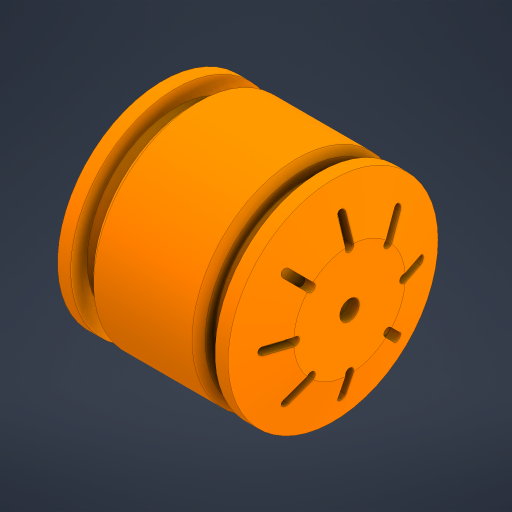
# Autodesk Inventor part: wheel
Saved by Autodesk Inventor 2024 (Build 280153000, 153)
## iProperties
Created: 2023-09-26
Part Number: wheel
Material: Типовые
Document SubType Name: Modeling
Designer: user
Density: 1 g/cm^3
Appearance: По умолчанию
Mass: 47.7551 g
Surface Area: 315.947 cm^2
Volume: 47.7551 cm^3
Author: user
Autodesk Inventor part; units mm, degrees
ref_plane "YZ Plane" through (0, 0, 0) normal (1, 0, 0) x (0, 1, 0)
ref_plane "XZ Plane" through (0, 0, 0) normal (0, 1, 0) x (-1, 0, 0)
sketch "Эскиз1" plane through (0, 0, 0) normal (0, 0, 1) x (1, 0, 0)
  line L0 (0, 0) -> (0, 32)
  line L1 (0, 32) -> (4, 32)
  line L2 (4, 32) -> (4, 27)
  line L3 (4, 27) -> (9, 27)
  line L4 (9, 27) -> (9, 32)
  line L5 (9, 32) -> (43, 32)
  line L6 (43, 32) -> (43, 27)
  line L7 (43, 27) -> (48, 27)
  line L8 (48, 27) -> (48, 32)
  line L9 (48, 32) -> (52, 32)
  line L10 (52, 32) -> (52, 0)
  line L11 (52, 0) -> (0, 0)
  dimension "d0" = 32
  dimension "d1" = 27
  dimension "d2" = 5
  dimension "d3" = 34
  dimension "d4" = 4
  constraints: 24 end point, 8 perpendicular, 6 point on line, 2 collinear, 1 vertical
  measures "d0" distance of L0.start L0.end
  measures "d1" vertical distance of L0.start L2.end
  measures "d2" distance of L2.end L3.end
  measures "d3" distance of L4.end L5.end
  measures "d4" distance of L0.end L1.end
revolve "Вращение1" add sketch "Эскиз1" angle 360 about axis through (52, 0, 0) along (-1, 0, 0)
sketch "Эскиз2" plane through (0, 0, 0) normal (0, 0, 1) x (1, 0, 0)
  line L0 (52, 32) -> (52, -32) projected
  line L1 (52, 32) -> (57, 17)
  line L2 (52, 0) -> (57, 0)
  line L3 (57, 0) -> (57, 17)
  point P0 (0, 0)
  dimension "d6" = 17
  dimension "d7" = 5
  constraints: 6 end point, 1 horizontal, 1 midpoint, 1 perpendicular
  measures "d6" distance of L2.end L1.end
  measures "d7" distance of L2.start L2.end
revolve "Вращение2" add sketch "Эскиз2" angle 360 about axis through (52, 0, 0) along (1, 0, 0)
shell "Оболочка1" thickness 3 removed faces 1 at (0, 9.4449, -4.957)
ref_plane "РабПлоскость1" through (26, 0, -32) normal (0, 0, 1) x (1, 0, 0)
chamfer "Фаска1" distance 2 angle 45 2 edges at (9, -32, 0) (43, -32, 0)
sketch "Эскиз9" plane through (57, 0, 0) normal (1, 0, 0) x (0, 0, -1)
  circle A0 centre (0, 0) radius 3
  dimension "d68" = 6
  constraints: 1 centre point, 1 coincident
  measures "d68" diameter of A0
extrude "Выдавливание6" cut sketch "Эскиз9" against normal through all
sketch "Эскиз21" plane through (54, 0, 0) normal (-1, 0, 0) x (0, 0, 1)
  circle A0 centre (0, 0) radius 3 projected
  circle A1 centre (0, 0) radius 16.5132 projected
extrude "Выдавливание17" add sketch "Эскиз21" along normal blind 0.1
sketch "Эскиз22" plane through (53.9, 0, 0) normal (-1, 0, 0) x (0, 0, 1)
  line L0 (-3.4641, -6) -> (3.4641, -6) projected
  line L1 (3.4641, -6) -> (6.9282, 0) projected
  line L2 (6.9282, 0) -> (3.4641, 6) projected
  line L3 (3.4641, 6) -> (-3.4641, 6) projected
  line L4 (-3.4641, 6) -> (-6.9282, 0) projected
  line L5 (-6.9282, 0) -> (-3.4641, -6) projected
  line L6 (6.3509, -11) -> (-6.3509, -11)
  line L7 (-6.3509, -11) -> (-12.7017, 0)
  line L8 (-12.7017, 0) -> (-6.3509, 11)
  line L9 (-6.3509, 11) -> (6.3509, 11)
  line L10 (6.3509, 11) -> (12.7017, 0)
  line L11 (12.7017, 0) -> (6.3509, -11)
  point P0 (0, 0)
  dimension "d121" = 5
  constraints: 12 end point, 5 other
  measures "d121" distance between parallel lines of L6 L0
extrude "Выдавливание18" add sketch "Эскиз22" along normal blind 14.75
sketch "Эскиз23" plane through (57, 0, 0) normal (1, 0, 0) x (0, 0, -1)
  line L0 (-12.7017, 0) -> (-6.3509, -11) construction
  circle A0 centre (0, 0) radius 16.5132 construction
  line L1 (-12.7017, 0) -> (-6.3509, -11) construction
  line L2 (-6.3509, -11) -> (6.3509, -11) construction
  line L3 (6.3509, -11) -> (12.7017, 0) construction
  line L4 (12.7017, 0) -> (6.3509, 11) construction
  line L5 (6.3509, 11) -> (-6.3509, 11) construction
  line L6 (-6.3509, 11) -> (-12.7017, 0) construction
  circle A1 centre (0, 0) radius 24 construction
  circle A2 centre (0, 0) radius 16.5132 projected
  line L7 (-16.5132, 0) -> (-24, 0) construction
  line L8 (-16.5132, 1.25) -> (-24, 1.25)
  line L9 (-24, -1.25) -> (-16.5132, -1.25)
  arc A3 (-16.5132, -1.25) -> (-16.5132, 1.25) centre (-16.5132, 0) ccw
  arc A4 (-24, 1.25) -> (-24, -1.25) centre (-24, 0) ccw
  point P0 (0, 0)
  point P1 (-20.2566, 0)
  dimension "d127" = 2.5
  constraints: 8 end point, 4 point on circle, 4 tangent, 3 horizontal alignment, 2 centre point, 1 horizontal, 1 midpoint, 1 parallel, 2 other
  measures "d127" distance of L8.start L9.end
extrude "Выдавливание19" cut sketch "Эскиз23" against normal blind 18.15 contours A3 A2 | A2 A3 L9 A4 L8 picked at (-16.0959, 0.049)
pattern_circular "Круговой массив4" count 8 over 360 about axis through (54.5, 0, 0) along (1, 0, 0) of "Выдавливание19"
